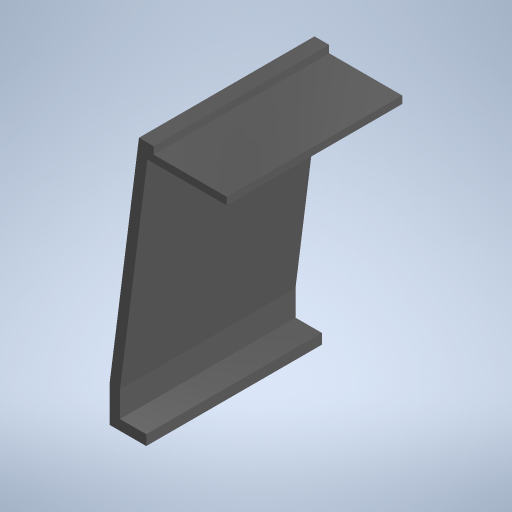
# Autodesk Inventor part: ROVER_carrozzeria_2
Saved by Autodesk Inventor 2023 (Build 270158000, 158)
## iProperties
Part Number: ROVER_carrozzeria_2
Material: Generico
Document SubType Name: Modellazione
Designer: aless
Appearance: Default
Author: aless
Autodesk Inventor part; units mm, degrees
ref_plane "Piano YZ" through (0, 0, 0) normal (1, 0, 0) x (0, 1, 0)
ref_plane "Piano XZ" through (0, 0, 0) normal (0, 1, 0) x (-1, 0, 0)
ref_plane "Piano XY" through (0, 0, 0) normal (0, 0, 1) x (1, 0, 0)
sketch "Schizzo1" plane through (0, 0, 0) normal (0, 0, 1) x (1, 0, 0)
  line L0 (25, 0) -> (0, 0)
  line L1 (0, 0) -> (0, 25)
  line L2 (0, 25) -> (20, 180)
  line L3 (20, 180) -> (30, 180)
  line L4 (30, 180) -> (30, 175)
  line L5 (30, 175) -> (80, 175)
  line L6 (80, 175) -> (80, 170)
  line L7 (80, 170) -> (25.7677, 170)
  line L8 (25.7677, 170) -> (7, 24.5503)
  line L9 (7, 24.5503) -> (7, 7)
  line L10 (7, 7) -> (25, 7)
  line L11 (25, 7) -> (25, 0)
  dimension "d0" = 7
  dimension "d1" = 7
  dimension "d2" = 7
  dimension "d3" = 10
  dimension "d4" = 5
  dimension "d5" = 25
  dimension "d6" = 180
  dimension "d7" = 10
  dimension "d8" = 50
  dimension "d9" = 20
  dimension "d10" = 25
  constraints: 24 end point, 6 perpendicular, 4 parallel, 1 horizontal
  measures "d0" distance of L10.end L0.start
  measures "d1" distance between parallel lines of L9 L1
  measures "d2" distance between parallel lines of L2 L8
  measures "d3" distance between parallel lines of L3 L7
  measures "d4" distance between parallel lines of L5 L7
  measures "d5" distance from line of L0.start L1
  measures "d6" distance between parallel lines of L3 L0
  measures "d7" distance of L2.end L3.end
  measures "d8" distance of L4.end L5.end
  measures "d9" distance from line of L1 L2.end
  measures "d10" distance of L0.end L1.end
extrude "Estrusione1" add sketch "Schizzo1" along normal blind 120
